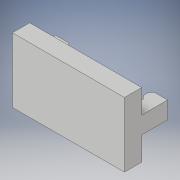
# Autodesk Inventor part: Cover
Saved by Autodesk Inventor 2019 (Build 230136000, 136)
## iProperties
Created: 2019-05-21
Part Number: Cover
Material: Generic
Document SubType Name: Modeling
Designer: aorfi
Density: 1 g/cm^3
Appearance: Default
Author: aorfi
Autodesk Inventor part; units mm, degrees
ref_plane "YZ Plane" through (0, 0, 0) normal (1, 0, 0) x (0, 1, 0)
ref_plane "XZ Plane" through (0, 0, 0) normal (0, 1, 0) x (-1, 0, 0)
ref_plane "XY Plane" through (0, 0, 0) normal (0, 0, 1) x (1, 0, 0)
sketch "Sketch2" plane through (0, 0, 0) normal (0, 0, 1) x (1, 0, 0)
  line L0 (-13, -7.5) -> (13, -7.5)
  line L1 (13, -7.5) -> (13, 7.5)
  line L2 (13, 7.5) -> (-13, 7.5)
  line L3 (-13, 7.5) -> (-13, -7.5)
  line L4 (-13, -7.5) -> (13, 7.5) construction
  line L5 (13, -7.5) -> (-13, 7.5) construction
  line L6 (-13, 2) -> (-10, 2)
  line L7 (-10, 2) -> (-10, -2)
  line L8 (-10, -2) -> (-13, -2)
  line L9 (0, 7.5) -> (0, -7.5) construction
  line L10 (13, -2) -> (10, -2)
  line L11 (10, -2) -> (10, 2)
  line L12 (10, 2) -> (13, 2)
  point P0 (0, 0)
  point P1 (0, 0)
  point P2 (-10, 0)
  point P3 (10, 0)
  dimension "d0" = 26
  dimension "d3" = 15
  dimension "d7" = 4
  dimension "d17" = 3
  constraints: 26 end point, 7 midpoint, 5 perpendicular, 4 point on line, 3 horizontal, 2 equal length, 2 horizontal alignment, 2 parallel
  measures "d0" distance of L2.end L1.end
  measures "d3" distance of L0.end L1.end
  measures "d7" distance of L6.end L7.end
  measures "d17" distance of L6.start L6.end
extrude "Extrusion1" add sketch "Sketch2" along normal mid plane 4
sketch "Sketch3" plane through (0, 0, -2) normal (0, 0, -1) x (-1, 0, 0)
  line L0 (-13, -7.5) -> (13, -7.5) projected
  line L1 (13, -7.5) -> (13, 7.5) projected
  line L2 (13, 7.5) -> (-13, 7.5) projected
  line L3 (-13, 7.5) -> (-13, -7.5) projected
  line L4 (-10, 5.5) -> (10, 5.5)
  line L5 (10, -5.5) -> (-10, -5.5)
  line L6 (-10, 5.5) -> (-10, -5.5)
  line L7 (10, 5.5) -> (10, -5.5)
  point P0 (0, 0)
  dimension "d4" = 2
  dimension "d18" = 2
  dimension "d19" = 3
  dimension "d20" = 3
  constraints: 8 end point, 1 parallel, 1 vertical
  measures "d4" distance between parallel lines of L2 L4
  measures "d18" distance between parallel lines of L0 L5
  measures "d19" distance between parallel lines of L3 L6
  measures "d20" distance between parallel lines of L1 L7
extrude "Extrusion2" cut sketch "Sketch3" against normal blind 2 contours L4 L7 L5 L6
extrude "Extrusion3" add sketch "Sketch2" along normal blind 2 and the other way blind 8 contours L3 L6 L7 L8 | L10 L11 L12 L1
sketch "Sketch4" plane through (13, 2, 2) normal (0, 1, 0) x (1, 0, 0)
  line L0 (-3, 4.007) -> (-3, 10)
  arc A0 (-3, 10) -> (-3, 7.4019) centre (-2.25, 8.701) ccw
  line L1 (-3, 7.4019) -> (-3, 10)
  line L2 (-13, 2) -> (-13, 0) construction
  line L3 (-26, 0) -> (0, 0) construction
  line L4 (-23, 10) -> (-23, 4.007)
  arc A1 (-23, 7.4019) -> (-23, 10) centre (-23.75, 8.701) ccw
  line L5 (-3, 4) -> (-3, 10) projected
  dimension "d13" = 1.5
  dimension "d14" = 0.75
  constraints: 8 end point, 4 point on circle, 4 symmetric about line, 2 centre point, 2 point on line, 1 collinear, 1 midpoint, 1 vertical, 1 other
  measures "d13" radius of A0
  measures "d14" distance from line of L0 A0.centre
extrude "Extrusion4" add sketch "Sketch4" against normal blind 4
equation "\"d18\" = d4"
equation "\"d20\" = d19"
body "Solid1"
